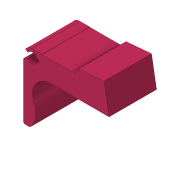
# Autodesk Inventor part: __VK_Stopper_Klinke
Saved by Autodesk Inventor 2025.1 (Build 291241000, 241)
## iProperties
Created: 2023-11-17
Part Number: __VK_Stopper_Klinke
Material: Generisch
Document SubType Name: Modeling
Designer: RP
Density: 1 g/cm^3
Appearance: Vorgabe(2)
Source: Unknown
Title: Stopper WT-240_Stoppstellung
Author: RP
Revision Number: ANY
Autodesk Inventor part; units mm, degrees
ref_plane "YZ Plane" through (0, 0, 0) normal (1, 0, 0) x (0, 1, 0)
ref_plane "XZ Plane" through (0, 0, 0) normal (0, 1, 0) x (-1, 0, 0)
ref_plane "XY Plane" through (0, 0, 0) normal (0, 0, 1) x (1, 0, 0)
sketch "Skizze2" plane through (0, 0, 0) normal (0, 0, 1) x (1, 0, 0)
  arc A0 (-10, -23.6564) -> (-24.8668, -44.0081) centre (-5.9511, -42.22) ccw
  line L0 (10, -23.22) -> (52.6, -23.22)
  line L1 (52.6, -23.22) -> (47.5218, 5.58)
  line L2 (47.5218, 5.58) -> (21.7421, 3.3246)
  line L3 (21.7421, 3.3246) -> (18.6, -0.42)
  line L4 (18.6, -2.22) -> (15.4, -2.22)
  line L5 (15.4, -2.22) -> (15.4, -2.42)
  line L6 (15.4, -2.42) -> (-15.1, -2.42)
  line L7 (-15.1, -2.42) -> (-15.1, -2.22)
  line L8 (-15.1, -2.22) -> (-25, -2.22)
  arc A1 (-25, -2.22) -> (-31.9282, -6.22) centre (-25, -10.22) ccw
  line L9 (-31.9282, -6.22) -> (-29.3301, -7.72)
  line L10 (-29.3301, -12.72) -> (-34, -15.4162)
  arc A2 (-20.2303, -8.72) -> (-29.3301, -7.72) centre (-25, -10.22) ccw
  arc A3 (-19.8, -11.72) -> (-19.8, -8.72) centre (-19.8, -10.22) ccw
  arc A4 (-29.3301, -12.72) -> (-20.2303, -11.72) centre (-25, -10.22) ccw
  line L11 (-20.2303, -8.72) -> (-19.8, -8.72)
  line L12 (-19.8, -11.72) -> (-20.2303, -11.72)
  line L13 (-34, -15.4162) -> (-34, -70.22)
  arc A5 (-34, -70.22) -> (-32, -72.22) centre (-32, -70.22) ccw
  line L14 (10, -23.22) -> (-5.9511, -23.22)
  arc A6 (-5.9511, -23.22) -> (-10, -23.6564) centre (-5.9511, -42.22) ccw
  line L15 (18.6, -0.42) -> (18.6, -2.22)
  arc A7 (-24.8668, -44.0081) -> (-24.0599, -46.9016) centre (-16.4084, -43.2085) ccw
  arc A8 (-29.0834, -72.22) -> (-25.7052, -70.4151) centre (-29.0834, -68.1561) ccw
  arc A9 (-25.7052, -70.4151) -> (-24.0599, -46.9016) centre (-45.4382, -57.22) ccw
  line L16 (-29.0834, -72.22) -> (-32, -72.22)
  point P0 (0, 0)
  point P1 (-21.7, -44.72)
  point P2 (-21.7, -75.72)
  point P3 (-21.7, -57.22)
  constraints: 34 end point, 21 point on circle, 10 centre point, 10 horizontal, 4 vertical, 3 tangent, 1 collinear, 1 concentric, 56 other
extrude "Extrusion2" add sketch "Skizze2" along normal mid plane 48
